Autodesk Fusion 360 part; units mm, degrees
note: some values were not read from the file. Set by a fixed rule: which sketch regions a step uses.
(part 2 of 2)
sketch "top" plane through (0, 0, 9) normal (0, 0, 1) x (1, 0, 0) in component "top_shell"
  circle A0 centre (5, 72) radius 1.75 construction
  circle A1 centre (42, 72) radius 1.75 construction
  circle A2 centre (5, 5) radius 1.75 construction
  circle A3 centre (42, 5) radius 1.75 construction
  line L0 (-0.5, -3.5) -> (47.5, -3.5)
  arc A4 (-3.5, -0.5) -> (-0.5, -3.5) centre (-0.5, -0.5) ccw
  line L1 (-3.5, 77.5) -> (-3.5, -0.5)
  arc A5 (47.5, -3.5) -> (50.5, -0.5) centre (47.5, -0.5) ccw
  line L2 (50.5, -0.5) -> (50.5, 77.5)
  line L3 (48.5, -0.5) -> (48.5, 77.5)
  line L4 (-0.5, -1.5) -> (47.5, -1.5)
  arc A6 (47.5, -1.5) -> (48.5, -0.5) centre (47.5, -0.5) ccw
  arc A7 (-1.5, -0.5) -> (-0.5, -1.5) centre (-0.5, -0.5) ccw
  line L5 (-1.5, 77.5) -> (-1.5, -0.5)
  arc A8 (-0.5, 80.5) -> (-3.5, 77.5) centre (-0.5, 77.5) ccw
  arc A9 (-0.5, 78.5) -> (-1.5, 77.5) centre (-0.5, 77.5) ccw
  line L6 (47.5, 78.5) -> (-0.5, 78.5)
  line L7 (47.5, 80.5) -> (-0.5, 80.5)
  arc A10 (48.5, 77.5) -> (47.5, 78.5) centre (47.5, 77.5) ccw
  arc A11 (50.5, 77.5) -> (47.5, 80.5) centre (47.5, 77.5) ccw
  line L8 (10.9538, 9.54) -> (9.525, 9.54) construction
  line L9 (10.9538, 67.96) -> (10.9538, 9.54) construction
  line L10 (9.525, 9.54) -> (8.0963, 9.54) construction
  line L11 (8.0963, 9.54) -> (1.7462, 9.54) construction
  line L12 (1.7462, 9.54) -> (1.7462, 36.6862) construction
  line L13 (1.7462, 36.6862) -> (1.7462, 40.8138) construction
  line L14 (1.7462, 40.8138) -> (1.7462, 62.0863) construction
  line L15 (9.525, 67.96) -> (10.9538, 67.96) construction
  line L16 (8.0963, 67.96) -> (9.525, 67.96) construction
  line L17 (1.7462, 67.96) -> (8.0963, 67.96) construction
  line L18 (1.7462, 63.6738) -> (1.7462, 67.96) construction
  line L19 (30.7975, 15.7163) -> (30.7975, 11.9063) construction
  line L20 (28.8925, 16.3513) -> (30.1625, 16.3513) construction
  line L21 (23.1775, 11.2713) -> (25.0825, 11.2713) construction
  line L22 (23.1775, 11.9063) -> (23.1775, 15.7163) construction
  line L23 (23.1775, 11.9063) -> (23.1775, 11.2713) construction
  line L24 (23.8125, 16.3513) -> (25.0825, 16.3513) construction
  line L25 (28.8925, 11.2713) -> (30.1625, 11.2713) construction
  circle A12 centre (40, 54) radius 1.5 construction
  circle A13 centre (23, 65) radius 1.4 construction
  line L26 (42.4498, 19.7168) -> (45.7518, 19.7168) construction
  line L27 (39.1478, 19.7168) -> (42.4498, 19.7168) construction
  line L28 (35.8458, 19.7168) -> (39.1478, 19.7168) construction
  line L29 (35.8458, 33.9408) -> (35.8458, 19.7168) construction
  line L30 (39.1478, 33.9408) -> (35.8458, 33.9408) construction
  line L31 (42.4498, 33.9408) -> (39.1478, 33.9408) construction
  line L32 (45.7518, 33.9408) -> (42.4498, 33.9408) construction
  line L33 (45.7518, 19.7168) -> (45.7518, 33.9408) construction
  line L34 (22.6775, 16.8513) -> (31.2975, 16.8513)
  line L35 (31.2975, 16.8513) -> (31.2975, 10.7713)
  line L36 (31.2975, 10.7713) -> (22.6775, 10.7713)
  line L37 (22.6775, 10.7713) -> (22.6775, 16.8513)
  line L38 (35.3458, 34.4408) -> (46.2518, 34.4408)
  line L39 (46.2518, 34.4408) -> (46.2518, 19.2168)
  line L40 (46.2518, 19.2168) -> (35.3458, 19.2168)
  line L41 (35.3458, 19.2168) -> (35.3458, 34.4408)
  line L42 (11.4538, 68.46) -> (1.2462, 68.46)
  line L43 (1.2462, 68.46) -> (1.2462, 9.04)
  line L44 (1.2462, 9.04) -> (11.4538, 9.04)
  line L45 (11.4538, 9.04) -> (11.4538, 68.46)
  circle A14 centre (23, 65) radius 2
  circle A15 centre (40, 54) radius 2
  line L46 (47.5, 79.7) -> (-0.5, 79.7)
  arc A16 (-0.5, 79.7) -> (-2.7, 77.5) centre (-0.5, 77.5) ccw
  line L47 (-2.7, 77.5) -> (-2.7, -0.5)
  arc A17 (-2.7, -0.5) -> (-0.5, -2.7) centre (-0.5, -0.5) ccw
  line L48 (-0.5, -2.7) -> (47.5, -2.7)
  arc A18 (47.5, -2.7) -> (49.7, -0.5) centre (47.5, -0.5) ccw
  line L49 (49.7, -0.5) -> (49.7, 77.5)
  arc A19 (49.7, 77.5) -> (47.5, 79.7) centre (47.5, 77.5) ccw
  circle A20 centre (5, 72) radius 1.25
  circle A21 centre (5, 72) radius 3
  circle A22 centre (42, 72) radius 1.25
  circle A23 centre (42, 72) radius 3
  circle A24 centre (42, 5) radius 1.25
  circle A25 centre (42, 5) radius 3
  circle A26 centre (5, 5) radius 1.25
  circle A27 centre (5, 5) radius 3
  line L50 (28.6703, 53.848) -> (15.4623, 53.848) construction
  line L51 (15.4623, 18.542) -> (15.4623, 53.848) construction
  line L52 (28.6703, 18.542) -> (28.6703, 53.848) construction
  line L53 (15.4623, 18.542) -> (20.7963, 18.542) construction
  line L54 (23.3362, 18.542) -> (28.6703, 18.542) construction
  line L55 (35.687, 9.398) -> (16.383, 9.398) construction
  line L56 (16.383, 9.398) -> (16.383, 7.366) construction
  arc A28 (23.3363, 18.542) -> (20.7963, 18.542) centre (22.0663, 18.542) ccw construction
  arc A29 (16.383, 5.334) -> (16.383, 7.366) centre (16.383, 6.35) ccw construction
  line L57 (16.383, 3.302) -> (16.383, 5.334) construction
  line L58 (16.383, 3.302) -> (35.687, 3.302) construction
  line L59 (35.687, 9.398) -> (35.687, 3.302) construction
  line L60 (15.4623, 54.348) -> (28.6703, 54.348)
  line L61 (29.1703, 53.848) -> (29.1703, 18.542)
  line L62 (28.6703, 18.042) -> (15.4623, 18.042)
  line L63 (14.9623, 18.542) -> (14.9623, 53.848)
  line L64 (16.383, 9.898) -> (35.687, 9.898)
  line L65 (36.187, 9.398) -> (36.187, 3.302)
  line L66 (35.687, 2.802) -> (16.383, 2.802)
  line L67 (15.883, 3.302) -> (15.883, 9.398)
  arc A30 (15.4623, 54.348) -> (14.9623, 53.848) centre (15.4623, 53.848) ccw
  arc A31 (29.1703, 53.848) -> (28.6703, 54.348) centre (28.6703, 53.848) ccw
  arc A32 (28.6703, 18.042) -> (29.1703, 18.542) centre (28.6703, 18.542) ccw
  arc A33 (14.9623, 18.542) -> (15.4623, 18.042) centre (15.4623, 18.542) ccw
  arc A34 (15.883, 3.302) -> (16.383, 2.802) centre (16.383, 3.302) ccw
  arc A35 (16.383, 9.898) -> (15.883, 9.398) centre (16.383, 9.398) ccw
  arc A36 (36.187, 9.398) -> (35.687, 9.898) centre (35.687, 9.398) ccw
  arc A37 (35.687, 2.802) -> (36.187, 3.302) centre (35.687, 3.302) ccw
  point P0 (47.5, -0.5)
  dimension "d82" = 0.5
  dimension "d83" = 0.5
  dimension "d84" = 0.5
  dimension "d85" = 0.5
  dimension "d86" = 0.5
  dimension "d87" = 0.5
  dimension "d88" = 0.5
  dimension "d89" = 0.5
  dimension "d90" = 0.5
  dimension "d91" = 0.5
  dimension "d92" = 0.5
  dimension "d93" = 0.5
  dimension "d94" = 4
  dimension "d95" = 4
  dimension "d96" = 1.2
  dimension "d99" = 2.5
  dimension "d100" = 6
  dimension "d101" = 2.5
  dimension "d102" = 6
  dimension "d103" = 2.5
  dimension "d104" = 6
  dimension "d105" = 2.5
  dimension "d106" = 6
  dimension "d117" = 0.5
  dimension "d118" = 0.5
  dimension "d119" = 0.5
  dimension "d120" = 0.5
  dimension "d121" = 0.5
  dimension "d122" = 0.5
  dimension "d123" = 0.5
  dimension "d124" = 0.5
  dimension "d125" = 0.5
  constraint horizontal L34
  constraint vertical L35
  constraint horizontal L36
  constraint vertical L37
  constraint horizontal L38
  constraint vertical L39
  constraint horizontal L40
  constraint vertical L41
  constraint horizontal L42
  constraint vertical L43
  constraint horizontal L44
  constraint vertical L45
  constraint concentric A13 A14
  constraint concentric A12 A15
  constraint concentric A0 A20
  constraint concentric A0 A21
  constraint concentric A1 A22
  constraint concentric A1 A23
  constraint concentric A3 A24
  constraint concentric A24 A25
  constraint concentric A2 A26
  constraint concentric A2 A27
  constraint horizontal L60
  constraint vertical L61
  constraint horizontal L62
  constraint vertical L63
  constraint horizontal L64
  constraint vertical L65
  constraint horizontal L66
  constraint vertical L67
  constraint tangent L60 A30
  constraint tangent L63 A30
  constraint tangent L60 A31
  constraint tangent L61 A31
  constraint equal A30 A31
  constraint tangent L61 A32
  constraint tangent L62 A32
  constraint equal A30 A32
  constraint tangent L62 A33
  constraint tangent L63 A33
  constraint equal A30 A33
  constraint tangent L66 A34
  constraint tangent L67 A34
  constraint equal A30 A34
  constraint tangent L64 A35
  constraint tangent L67 A35
  constraint equal A30 A35
  constraint tangent L64 A36
  constraint tangent L65 A36
  constraint equal A30 A36
  constraint tangent L65 A37
  constraint tangent L66 A37
  constraint equal A30 A37
  measures "d82" distance of L24 L34
  measures "d83" distance of L21 L36
  measures "d84" distance of L22 L37
  measures "d85" distance of L19 L35
  measures "d86" distance of L30 L38
  measures "d87" distance of L28 L40
  measures "d88" distance of L29 L41
  measures "d89" distance of L33 L39
  measures "d90" distance of L9 L45
  measures "d91" distance of L12 L43
  measures "d92" distance of L11 L44
  measures "d93" distance of L17 L42
  measures "d94" diameter of A14
  measures "d95" diameter of A15
  measures "d99" diameter of A20
  measures "d100" diameter of A21
  measures "d101" diameter of A22
  measures "d102" diameter of A23
  measures "d103" diameter of A24
  measures "d104" diameter of A25
  measures "d105" diameter of A26
  measures "d106" diameter of A27
  measures "d117" distance of L50 L60
  measures "d118" distance of L52 L61
  measures "d119" distance of L51 L63
  measures "d120" distance of L53 L62
  measures "d121" distance of L55 L64
  measures "d122" distance of L58 L66
  measures "d123" distance of L57 L67
  measures "d124" distance of L59 L65
  measures "d125" radius of A30
extrude "Extrude1''" add sketch "top" along normal blind 2 separate body contours L0 A4 L1 A5 L2 A8 L7 A11 | L3 L4 A6 A7 L5 A9 L6 A10 | L46 A16 L47 A17 L48 A18 L49 A19 | A20 | A21 | A22 | A23 | A24 | A25 | A26 | A27 | L60 L61 L62 L63 A30 A31 A32 A33 | L64 L65 L66 L67 A34 A35 A36 A37 makes body 3 in component "top_shell"
extrude "Extrude2''" add sketch "top" against normal blind 2.5 contours L0 A4 L1 A5 L2 A8 L7 A11 bodies 3 in component "top_shell"
extrude "Extrude3''" add sketch "top" against normal blind 1 contours L46 A16 L47 A17 L48 A18 L49 A19 bodies 3 in component "top_shell"
extrude "Extrude4''" add sketch "top" against normal blind 9 contours A21 | A23 | A25 | A27 bodies 3 in component "top_shell"
fillet "Fillet1''" radius 2 8 edges at (23.5, 80.5, 11) (-2.6213, 79.6213, 11) (-3.5, 38.5, 11) (-2.6213, -2.6213, 11) (23.5, -3.5, 11) (49.6213, -2.6213, 11) (50.5, 38.5, 11) (49.6213, 79.6213, 11) on bodies 3 in component "top_shell"
extrude "Extrude5'" cut sketch "top" along normal blind 1 contours L60 L61 L62 L63 A30 A31 A32 A33 | L64 L65 L66 L67 A34 A35 A36 A37 bodies 3 in component "top_shell"
component "PCB" placed x (1, 0, 0) y (0, 1, 0) z (0, 0, 1) at (0, 0, 0)
component "bottom_shell" placed x (1, 0, 0) y (0, 1, 0) z (0, 0, 1) at (0, 0, 0)
component "top_shell" placed x (1, 0, 0) y (0, 1, 0) z (0, 0, 1) at (0, 0, 0)
equation "wall = 2 mm"
equation "below = 3 mm"
equation "above = 9 mm"
equation "wall_distance = 1.5 mm"
equation "d39 = -below - 1.6 mm"
equation "inner_radius = 1 mm"
equation "d42 = inner_radius"
equation "d43 = wall * 0.4"
equation "d44 = wall"
equation "bottom_drill = 3.5 mm"
equation "bottom_screw = 6 mm"
equation "bottom_post = 10 mm"
equation "d48 = bottom_drill"
equation "d49 = bottom_screw"
equation "d50 = bottom_post"
equation "d51 = bottom_drill"
equation "d52 = bottom_screw"
equation "d53 = bottom_post"
equation "d54 = bottom_post"
equation "d55 = bottom_screw"
equation "d56 = bottom_drill"
equation "d57 = bottom_drill"
equation "d58 = bottom_screw"
equation "d59 = bottom_post"
equation "d60 = -wall"
equation "d62 = below"
equation "overlap = 1.5 mm"
equation "top_height = wall + overlap + 1 mm"
equation "pcb = 1.6 mm"
equation "total_height = above + pcb + below + 2 * wall"
equation "bottom_height = total_height - top_height"
equation "d71 = bottom_height - wall"
equation "d73 = bottom_height - wall + overlap"
equation "fillet = 2 mm"
equation "d77 = fillet"
equation "d80 = above"
equation "cutout_distance = 0.5 mm"
equation "d82 = cutout_distance"
equation "d83 = cutout_distance"
equation "d84 = cutout_distance"
equation "d85 = cutout_distance"
equation "d86 = cutout_distance"
equation "d87 = cutout_distance"
equation "d88 = cutout_distance"
equation "d89 = cutout_distance"
equation "d90 = cutout_distance"
equation "d91 = cutout_distance"
equation "d92 = cutout_distance"
equation "d93 = cutout_distance"
equation "d95 = d94"
equation "d96 = wall * 0.6"
equation "top_post = 6 mm"
equation "top_drill = 2.5 mm"
equation "d99 = top_drill"
equation "d100 = top_post"
equation "d101 = top_drill"
equation "d102 = top_post"
equation "d103 = top_drill"
equation "d104 = top_post"
equation "d105 = top_drill"
equation "d106 = top_post"
equation "d107 = wall"
equation "d109 = -top_height + wall"
equation "d111 = -top_height + wall + overlap"
equation "d113 = -above"
equation "d116 = fillet"
equation "d117 = cutout_distance"
equation "d118 = cutout_distance"
equation "d119 = cutout_distance"
equation "d120 = cutout_distance"
equation "d121 = cutout_distance"
equation "d122 = cutout_distance"
equation "d123 = cutout_distance"
equation "d124 = cutout_distance"
equation "d125 = cutout_distance"
equation "ic_indent = 1 mm"
equation "d127 = ic_indent"
named bodies: "pcb", "bottom_shell", "top_shell"
